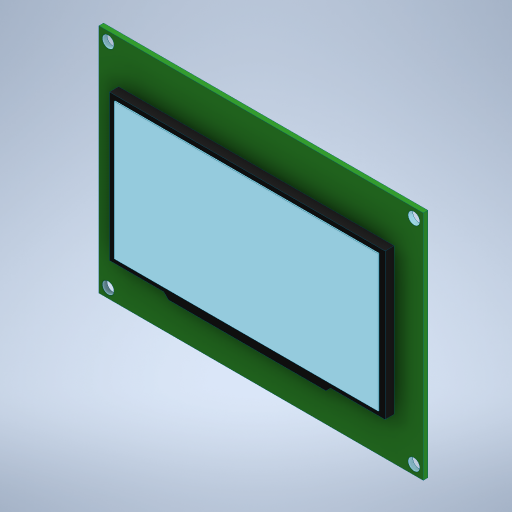
# Autodesk Inventor part: Adafruit 2.4 OLED display
Saved by Autodesk Inventor 2023 (Build 270158000, 158)
## iProperties
Created: 2022-05-21
Part Number: Adafruit 2.4 OLED display
Material: Generic
Document SubType Name: Modeling
Designer: Jochen
Density: 1 g/cm^3
Appearance: Default
Author: Jochen
Autodesk Inventor part; units mm, degrees
ref_plane "YZ Plane" through (0, 0, 0) normal (1, 0, 0) x (0, 1, 0)
ref_plane "XZ Plane" through (0, 0, 0) normal (0, 1, 0) x (-1, 0, 0)
ref_plane "XY Plane" through (0, 0, 0) normal (0, 0, 1) x (1, 0, 0)
sketch "Sketch1" plane through (0, 0, 0) normal (0, 0, 1) x (1, 0, 0)
  line L0 (-27.505, 13.7) -> (27.505, 13.7)
  line L1 (27.505, 13.7) -> (27.505, -13.7)
  line L2 (27.505, -13.7) -> (-27.505, -13.7)
  line L3 (-27.505, -13.7) -> (-27.505, 13.7)
  line L4 (-49, 0) -> (49, 0) construction
  line L5 (0, -36) -> (0, 34) construction
  line L6 (-28.505, 14.745) -> (28.505, 14.745)
  line L7 (28.505, 14.745) -> (28.505, -14.745)
  line L8 (28.505, -14.745) -> (-28.505, -14.745)
  line L9 (-28.505, -14.745) -> (-28.505, 14.745)
  line L10 (-29.75, 15.75) -> (29.75, 15.75)
  line L11 (29.75, 15.75) -> (29.75, -15.75)
  line L12 (-29.75, -15.75) -> (-29.75, 15.75)
  line L13 (-31, 17) -> (31, 17)
  line L14 (31, 17) -> (31, -22)
  line L15 (31, -22) -> (-31, -22)
  line L16 (-31, -22) -> (-31, 17)
  line L17 (-31, 17) -> (-29.75, 15.75) construction
  line L18 (-18, -15.75) -> (-17, -16.75)
  line L19 (-17, -16.75) -> (17, -16.75)
  line L20 (17, -16.75) -> (18, -15.75)
  line L21 (29.75, -15.75) -> (18, -15.75)
  line L22 (-18, -15.75) -> (-29.75, -15.75)
  line L23 (-35, 24) -> (35, 24)
  line L24 (35, 24) -> (35, -26)
  line L25 (35, -26) -> (-35, -26)
  line L26 (-35, -26) -> (-35, 24)
  line L27 (-35, -26) -> (-31, -22) construction
  circle A0 centre (-33, -24) radius 1.25
  circle A1 centre (-33, 22) radius 1.25
  circle A2 centre (33, -24) radius 1.25
  circle A3 centre (33, 22) radius 1.25
  point P0 (0, 0)
  dimension "d0" = 55.01
  dimension "d1" = 27.4
  dimension "d2" = 57.01
  dimension "d3" = 29.49
  dimension "d4" = 59.5
  dimension "d5" = 31.5
  dimension "d6" = 62
  dimension "d7" = 39
  dimension "d8" = 34
  dimension "d10" = 1
  dimension "d11" = 70
  dimension "d12" = 50
  dimension "d21" = 2
  dimension "d22" = 2.5
  dimension "d33" = 46
  dimension "d36" = 66
  constraints: 52 end point, 11 parallel, 7 horizontal, 6 perpendicular, 4 centre point, 1 collinear, 1 midpoint, 1 vertical, 17 other
  measures "d0" distance of L1.end L2.end
  measures "d1" distance of L2.end L0.start
  measures "d2" distance of L6.start L6.end
  measures "d3" distance of L8.end L6.start
  measures "d4" distance of L10.start L10.end
  measures "d5" distance of L12.start L10.start
  measures "d6" distance of L13.start L13.end
  measures "d7" distance of L15.end L13.start
  measures "d8" distance of L18.end L19.end
  measures "d10" distance between parallel lines of L19 L22
  measures "d11" distance of L23.start L23.end
  measures "d12" distance of L25.end L23.start
  measures "d21" distance from line of L26 A0.centre
  measures "d22" diameter of A0
  measures "d33" distance of A0.centre A1.centre
  measures "d36" distance of A0.centre A2.centre
extrude "Extrusion1" add sketch "Sketch1" along normal blind 1 contours L0 L1 L2 L3 | L6 L7 L8 L9 | L10 L11 L21 L20 L19 L18 L22 L12 | L13 L14 L15 L16 | L23 L24 L25 L26
extrude "Extrusion2" add sketch "Sketch1" along normal blind 2 contours L0 L1 L2 L3
extrude "Extrusion3" add sketch "Sketch1" along normal blind 2 from surface at 2 contours L0 L1 L2 L3 | L6 L7 L8 L9 | L10 L11 L21 L20 L19 L18 L22 L12
extrude "Extrusion4" add sketch "Sketch1" along normal blind 0.2 from surface at 4 contours L0 L1 L2 L3 | L6 L7 L8 L9
equation "\"d33\" = d12 - 2 * d21"
equation "\"d36\" = d11 - 2 * d21"
body "Solid1"
